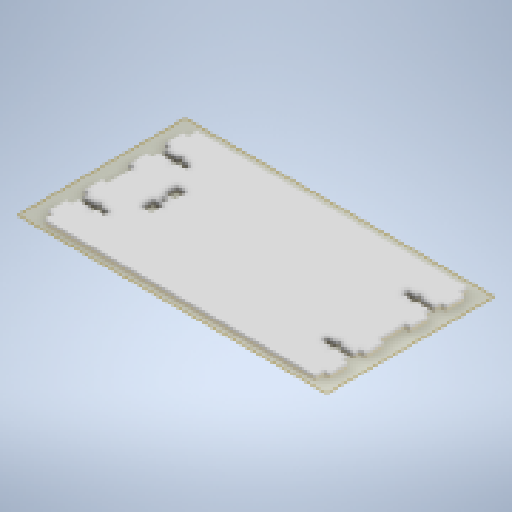
# Autodesk Inventor part: Нижняя часть головы
Saved by Autodesk Inventor 2023.2 (Build 272271030, 271C)
## iProperties
Created: 2024-02-16
Part Number: Нижняя часть головы
Material: Типовые
Document SubType Name: Modeling
Designer: I9232
Density: 1 g/cm^3
Appearance: По умолчанию
Author: I9232
Autodesk Inventor part; units mm, degrees
ref_plane "YZ Plane" through (0, 0, 0) normal (1, 0, 0) x (0, 1, 0)
ref_plane "XY Plane" through (0, 0, 0) normal (0, 0, 1) x (1, 0, 0)
sketch "Эскиз1" plane through (0, 0, 0) normal (0, 1, 0) x (-1, 0, 0)
  line L0 (75.318, 42.5) -> (-75.318, 42.5)
  line L1 (-75.318, 42.5) -> (-75.318, -42.5)
  line L2 (-75.318, -42.5) -> (75.318, -42.5)
  line L3 (75.318, -42.5) -> (75.318, 42.5)
  line L4 (75.318, 42.5) -> (-75.318, -42.5) construction
  line L5 (-75.318, 42.5) -> (75.318, -42.5) construction
  point P0 (0, 0)
  dimension "d0" = 150.636
  dimension "d1" = 85
  constraints: 12 end point, 2 midpoint, 2 parallel, 1 horizontal, 1 perpendicular
  measures "d0" distance of L1.end L2.end
  measures "d1" distance of L2.end L0.start
extrude "Выдавливание1" add sketch "Эскиз1" along normal mid plane 3
sketch "Эскиз3" plane through (-75.318, -1.5, 42.5) normal (-1, 0, 0) x (0, 0, 1)
  line L0 (-85, 0) -> (0, 0) projected
  line L1 (-80, 3) -> (-70, 3)
  line L2 (-70, 3) -> (-70, 0)
  line L3 (-70, 0) -> (-80, 0)
  line L4 (-80, 0) -> (-80, 3)
  line L5 (-80, 3) -> (-70, 0) construction
  line L6 (-70, 3) -> (-80, 0) construction
  line L7 (-60, 3) -> (-50, 3)
  line L8 (-50, 3) -> (-50, 0)
  line L9 (-50, 0) -> (-60, 0)
  line L10 (-60, 0) -> (-60, 3)
  line L11 (-60, 3) -> (-50, 0) construction
  line L12 (-50, 3) -> (-60, 0) construction
  line L13 (-35, 3) -> (-25, 3)
  line L14 (-25, 3) -> (-25, 0)
  line L15 (-25, 0) -> (-35, 0)
  line L16 (-35, 0) -> (-35, 3)
  line L17 (-35, 3) -> (-25, 0) construction
  line L18 (-25, 3) -> (-35, 0) construction
  line L19 (-15, 3) -> (-5, 3)
  line L20 (-5, 3) -> (-5, 0)
  line L21 (-5, 0) -> (-15, 0)
  line L22 (-15, 0) -> (-15, 3)
  line L23 (-15, 3) -> (-5, 0) construction
  line L24 (-5, 3) -> (-15, 0) construction
  line L25 (0, 0) -> (0, 3) projected
  line L26 (-85, 0) -> (-85, 3) projected
  point P0 (-42.5, 1.5)
  point P1 (-75, 1.5)
  point P2 (-55, 1.5)
  point P3 (-30, 1.5)
  point P4 (-10, 1.5)
  point P5 (-15, 1.5)
  point P6 (-25, 1.5)
  point P7 (-60, 1.5)
  point P8 (-35, 0)
  point P9 (-15, 0)
  dimension "d8" = 10
  dimension "d9" = 10
  dimension "d10" = 10
  dimension "d11" = 10
  dimension "d12" = 3
  dimension "d13" = 10
  dimension "d14" = 10
  dimension "d15" = 5
  dimension "d16" = 5
  constraints: 48 end point, 11 midpoint, 11 parallel, 4 horizontal, 4 perpendicular, 4 point on line
  measures "d8" distance of L1.start L1.end
  measures "d9" distance of L7.start L7.end
  measures "d10" distance of L13.start L13.end
  measures "d11" distance of L19.start L19.end
  measures "d12" distance of L7.end L8.end
  measures "d13" distance of point (-15, 1.5) point (-25, 1.5)
  measures "d14" distance from line of point (-60, 1.5) L2
  measures "d15" distance between parallel lines of L25 L20
  measures "d16" distance between parallel lines of L26 L4
extrude "Выдавливание3" add sketch "Эскиз3" along normal blind 3
sketch "Эскиз4" plane through (75.318, -1.5, -42.5) normal (1, 0, 0) x (0, 0, -1)
  line L0 (-85, 3) -> (0, 3) projected
  line L1 (-80, 0.0026) -> (-70, 0.0026)
  line L2 (-70, 0.0026) -> (-70, 3)
  line L3 (-70, 3) -> (-80, 3)
  line L4 (-80, 3) -> (-80, 0.0026)
  line L5 (-80, 0.0026) -> (-70, 3) construction
  line L6 (-70, 0.0026) -> (-80, 3) construction
  line L7 (-60, 0.0026) -> (-50, 0.0026)
  line L8 (-50, 0.0026) -> (-50, 3)
  line L9 (-50, 3) -> (-60, 3)
  line L10 (-60, 3) -> (-60, 0.0026)
  line L11 (-60, 0.0026) -> (-50, 3) construction
  line L12 (-50, 0.0026) -> (-60, 3) construction
  line L13 (-42.5, 3) -> (-42.5, 0) construction
  line L14 (0, 0) -> (-85, 0) projected
  line L15 (-5, 0.0026) -> (-15, 0.0026)
  line L16 (-15, 0.0026) -> (-15, 3)
  line L17 (-15, 3) -> (-5, 3)
  line L18 (-5, 3) -> (-5, 0.0026)
  line L19 (-5, 0.0026) -> (-15, 3) construction
  line L20 (-15, 0.0026) -> (-5, 3) construction
  line L21 (-25, 0.0026) -> (-35, 0.0026)
  line L22 (-35, 0.0026) -> (-35, 3)
  line L23 (-35, 3) -> (-25, 3)
  line L24 (-25, 3) -> (-25, 0.0026)
  line L25 (-25, 0.0026) -> (-35, 3) construction
  line L26 (-35, 0.0026) -> (-25, 3) construction
  line L27 (-85, 3) -> (-85, 0) projected
  point P0 (-42.5, 1.5)
  point P1 (-75, 1.5013)
  point P2 (-55, 1.5013)
  point P3 (-10, 1.5013)
  point P4 (-30, 1.5013)
  point P5 (-35, 3)
  point P6 (-5, 3)
  point P7 (-15, 3)
  dimension "d19" = 10
  dimension "d24" = 20
  dimension "d29" = 5
  constraints: 50 end point, 10 symmetric about line, 3 midpoint, 2 horizontal, 2 parallel, 1 perpendicular, 1 point on line, 13 other
  measures "d19" distance of L1.start L1.end
  measures "d24" distance of L1.start L7.start
  measures "d29" distance between parallel lines of L27 L4
extrude "Выдавливание4" add sketch "Эскиз4" along normal blind 3
sketch "Эскиз5" plane through (0, 1.5, 0) normal (0, 1, 0) x (1, 0, 0)
  line L0 (-75.318, 7.5) -> (-75.318, -7.5) projected
  line L1 (-54.4999, -2.8628) -> (-54.4999, -9.8628)
  line L2 (-54.4999, -9.8628) -> (-48.4999, -9.8628)
  line L3 (-48.4999, -9.8628) -> (-48.4999, -2.8628)
  line L4 (-48.4999, -2.8628) -> (-54.4999, -2.8628)
  line L5 (-48.4999, 3.1372) -> (-48.4999, 10.1372)
  line L6 (-48.4999, 10.1372) -> (-54.4999, 10.1372)
  line L7 (-54.4999, 10.1372) -> (-54.4999, 3.1372)
  line L8 (-54.4999, 3.1372) -> (-48.4999, 3.1372)
  line L9 (-51.4999, -2.8628) -> (-51.4999, 3.1372)
  circle A0 centre (-51.4999, 0.1372) radius 1.5
  point P0 (0, 0)
  dimension "d37" = 3
  constraints: 18 end point, 3 midpoint, 1 centre point
  measures "d37" diameter of A0
extrude "Выдавливание5" cut sketch "Эскиз5" against normal blind 3
sketch "Эскиз6" plane through (0, 1.5, 0) normal (0, 1, 0) x (1, 0, 0)
  line L0 (75.318, -27.5) -> (75.318, -17.5) projected
  line L1 (60.318, -24) -> (60.318, -21)
  line L2 (75.318, -21) -> (75.318, -24)
  line L3 (67.818, -25.55) -> (65.318, -25.55)
  line L4 (65.318, -19.45) -> (67.818, -19.45)
  line L5 (67.818, -19.45) -> (67.818, -21)
  line L6 (67.818, -24) -> (67.818, -25.55)
  line L7 (75.318, -24) -> (67.818, -24)
  line L8 (65.318, -24) -> (60.318, -24)
  line L9 (65.318, -25.55) -> (65.318, -24)
  line L10 (65.318, -21) -> (65.318, -19.45)
  line L11 (60.318, -21) -> (65.318, -21)
  line L12 (67.818, -21) -> (75.318, -21)
  line L13 (66.568, 0) -> (53.2147, 0) construction
  line L14 (0, -10.2584) -> (0, 8.5624) construction
  line L15 (75.318, 27.5) -> (75.318, 17.5)
  line L16 (60.318, 24) -> (60.318, 21)
  line L17 (75.318, 21) -> (75.318, 24)
  line L18 (67.818, 25.55) -> (65.318, 25.55)
  line L19 (65.318, 19.45) -> (67.818, 19.45)
  line L20 (67.818, 19.45) -> (67.818, 21)
  line L21 (67.818, 24) -> (67.818, 25.55)
  line L22 (75.318, 24) -> (67.818, 24)
  line L23 (65.318, 24) -> (60.318, 24)
  line L24 (65.318, 25.55) -> (65.318, 24)
  line L25 (65.318, 21) -> (65.318, 19.45)
  line L26 (60.318, 21) -> (65.318, 21)
  line L27 (67.818, 21) -> (75.318, 21)
  line L28 (0, 10.2584) -> (0, -8.5624) construction
  line L29 (-75.318, -27.5) -> (-75.318, -17.5)
  line L30 (-60.318, -24) -> (-60.318, -21)
  line L31 (-75.318, -21) -> (-75.318, -24)
  line L32 (-67.818, -25.55) -> (-65.318, -25.55)
  line L33 (-65.318, -19.45) -> (-67.818, -19.45)
  line L34 (-67.818, -19.45) -> (-67.818, -21)
  line L35 (-67.818, -24) -> (-67.818, -25.55)
  line L36 (-75.318, -24) -> (-67.818, -24)
  line L37 (-65.318, -24) -> (-60.318, -24)
  line L38 (-65.318, -25.55) -> (-65.318, -24)
  line L39 (-65.318, -21) -> (-65.318, -19.45)
  line L40 (-60.318, -21) -> (-65.318, -21)
  line L41 (-67.818, -21) -> (-75.318, -21)
  line L42 (-66.568, 0) -> (-53.2147, 0) construction
  line L43 (-60.318, 24) -> (-60.318, 21)
  line L44 (-65.318, 24) -> (-60.318, 24)
  line L45 (-60.318, 21) -> (-65.318, 21)
  line L46 (-65.318, 21) -> (-65.318, 19.45)
  line L47 (-65.318, 19.45) -> (-67.818, 19.45)
  line L48 (-67.818, 19.45) -> (-67.818, 21)
  line L49 (-65.318, 25.55) -> (-65.318, 24)
  line L50 (-67.818, 25.55) -> (-65.318, 25.55)
  line L51 (-67.818, 24) -> (-67.818, 25.55)
  line L52 (-67.818, 21) -> (-75.318, 21)
  line L53 (-75.318, 21) -> (-75.318, 24)
  line L54 (-75.318, 27.5) -> (-75.318, 17.5)
  line L55 (-75.318, 24) -> (-67.818, 24)
  point P0 (0, 0)
  point P1 (67.818, -23.3834)
  point P2 (67.818, 23.3834)
  point P3 (-67.818, -23.3834)
  point P4 (-67.818, 23.3834)
  point P5 (-75.318, -21)
  point P6 (75.318, -22.5)
  dimension "d38" = 6.1
  dimension "d39" = 3
  dimension "d40" = 2.5
  dimension "d41" = 15
  dimension "d42" = 1.55
  dimension "d43" = 1.55
  dimension "d44" = 1.55
  dimension "d45" = 1.55
  constraints: 110 end point, 49 symmetric about line, 10 parallel, 4 horizontal, 4 perpendicular, 4 point on line, 2 midpoint, 1 vertical
  measures "d38" distance of L3.end L4.start
  measures "d39" distance of L1.start L1.end
  measures "d40" distance of L3.start L3.end
  measures "d41" distance of L2.end L1.start
  measures "d42" distance of L3.end L8.start
  measures "d43" distance of L6.start L3.start
  measures "d44" distance of L4.end L5.end
  measures "d45" distance of L10.start L4.start
extrude "Выдавливание6" cut sketch "Эскиз6" against normal blind 3
